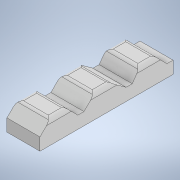
# Autodesk Inventor part: mould
Saved by Autodesk Inventor 2021 (Build 250183000, 183)
## iProperties
Created: 2021-07-01
Part Number: mould
Material: Generic
Document SubType Name: Modeling
Designer: HP
Density: 1 g/cm^3
Appearance: Default
Author: HP
Autodesk Inventor part; units mm, degrees
ref_plane "YZ Plane" through (0, 0, 0) normal (1, 0, 0) x (0, 1, 0)
ref_plane "XZ Plane" through (0, 0, 0) normal (0, 1, 0) x (-1, 0, 0)
ref_plane "XY Plane" through (0, 0, 0) normal (0, 0, 1) x (1, 0, 0)
sketch "Sketch4" plane through (0, 0, 0) normal (1, 0, 0) x (0, 1, 0)
  line L0 (88.8188, -396.6218) -> (88.8188, -1896.6218)
  line L1 (88.8188, -1896.6218) -> (238.8188, -1896.6218)
  line L2 (238.8188, -1896.6218) -> (238.8188, -1821.6218)
  line L3 (238.8188, -1821.6218) -> (367.6368, -1694.6481)
  line L4 (367.6368, -1694.6481) -> (367.6368, -1494.6481)
  line L5 (367.6368, -1494.6481) -> (238.8188, -1401.7722)
  line L6 (238.8188, -1401.7722) -> (238.8188, -1326.7722)
  line L7 (238.8188, -1326.7722) -> (367.6368, -1148.1032)
  line L8 (367.6368, -1148.1032) -> (367.6368, -948.1032)
  line L9 (367.6368, -948.1032) -> (238.8188, -817.4142)
  line L10 (238.8188, -817.4142) -> (238.8188, -742.4142)
  line L11 (238.8188, -742.4142) -> (367.6368, -615.4405)
  line L12 (367.6368, -615.4405) -> (367.6368, -415.4405)
  line L13 (367.6368, -415.4405) -> (238.8188, -284.7516)
  line L14 (238.8188, -284.7516) -> (88.8188, -284.7516)
  line L15 (88.8188, -284.7516) -> (88.8188, -396.6218)
  point P0 (0, 0)
  dimension "d47" = 1500
  dimension "d48" = 150
  dimension "d49" = 75
  dimension "d50" = 200
  dimension "d51" = 75
  dimension "d52" = 200
  dimension "d53" = 75
  dimension "d54" = 200
  constraints: 32 end point, 10 point on line, 7 perpendicular, 2 parallel, 1 vertical
  measures "d47" distance of L0.start L0.end
  measures "d48" distance of L0.end L1.end
  measures "d49" distance of L1.end L3.start
  measures "d50" distance of L3.end L5.start
  measures "d51" distance of L6.start L7.start
  measures "d52" distance of L8.start L8.end
  measures "d53" distance of L9.end L10.end
  measures "d54" distance of L11.end L12.end
extrude "Extrusion4" add sketch "Sketch4" along normal blind 400
fillet "Fillet5" radius 50 12 edges at (200, 367.6368, -415.4405) (400, 367.6368, -515.4405) (200, 367.6368, -615.4405) (200, 367.6368, -948.1032) (0, 367.6368, -515.4405) (0, 367.6368, -1048.1032) (200, 367.6368, -1148.1032) (400, 367.6368, -1048.1032) (200, 367.6368, -1494.6481) (400, 367.6368, -1594.6481) (200, 367.6368, -1694.6481) (0, 367.6368, -1594.6481)
body "Solid3"
